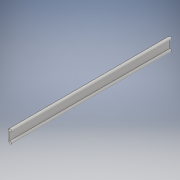
# Autodesk Inventor part: Linear Guide Rail Temporary
Saved by Autodesk Inventor 2018 (Build 220112000, 112)
## iProperties
Created: 2019-01-11
Part Number: Linear Guide Rail Temporary
Material: Generic
Document SubType Name: Modeling
Designer: s-2512711
Density: 1 g/cm^3
Appearance: Default
Author: s-2512711
Autodesk Inventor part; units mm, degrees
ref_plane "YZ Plane" through (0, 0, 0) normal (1, 0, 0) x (0, 1, 0)
ref_plane "XZ Plane" through (0, 0, 0) normal (0, 1, 0) x (-1, 0, 0)
ref_plane "XY Plane" through (0, 0, 0) normal (0, 0, 1) x (1, 0, 0)
sketch "Sketch1" plane through (0, 0, 0) normal (0, 0, 1) x (1, 0, 0)
  line L0 (0, 0) -> (5.461, 0)
  line L1 (5.461, 0) -> (5.461, 39.8272)
  line L2 (5.461, 39.8272) -> (0, 39.8272)
  line L3 (0, 39.8272) -> (0, 0)
  dimension "d0" = 5.461
  dimension "d1" = 39.8272
  constraints: 8 end point, 2 parallel, 1 horizontal, 1 perpendicular
  measures "d0" distance of L2.end L1.end
  measures "d1" distance of L1.end L0.end
extrude "Extrusion1" add sketch "Sketch1" along normal blind 609.6
sketch "Sketch2" plane through (0, 0, 609.6) normal (0, 0, 1) x (1, 0, 0)
  line L0 (5.461, 0) -> (5.461, 39.8272) projected
  line L1 (5.461, 0) -> (4.191, 0) construction
  line L2 (0, 0) -> (5.461, 0) projected
  line L3 (4.191, 0) -> (9.1821, 0) construction
  circle A0 centre (9.1821, 0) radius 4.9911
  line L4 (5.461, 19.9136) -> (0, 19.9136) construction
  line L5 (0, 39.8272) -> (0, 0) construction
  line L6 (5.461, 39.8272) -> (4.191, 39.8272) construction
  circle A1 centre (9.1821, 39.8272) radius 4.9911
  dimension "d4" = 1.27
  dimension "d5" = 4.9911
  constraints: 8 end point, 2 horizontal alignment, 2 midpoint, 2 point on line, 2 symmetric about line, 1 coincident, 1 horizontal, 4 other
  measures "d4" distance of L0.start L1.end
  measures "d5" distance of L1.end L3.end
extrude "Extrusion2" add sketch "Sketch2" against normal blind 609.6
body "Solid1"
